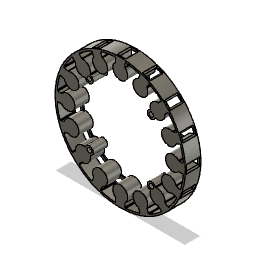
ball_syahei_20221011 v1 (Autodesk Fusion 360 design; units mm, degrees)
Autodesk Fusion 360 part; units mm, degrees
(part 1 of 2)
sketch "スケッチ1" plane through (0, 0, 0) normal (0, 0, 1) x (1, 0, 0)
  line L0 (-2.25, 51.3973) -> (-2.25, 46.9371)
  line L1 (2.25, 51.3973) -> (2.25, 46.9371)
  arc A0 (-2.6591, 46.1303) -> (2.6591, 46.1303) centre (0, 42.5) ccw
  arc A1 (2.25, 46.9371) -> (2.6591, 46.1303) centre (3.25, 46.9371) ccw
  arc A2 (-2.6591, 46.1303) -> (-2.25, 46.9371) centre (-3.25, 46.9371) ccw
  arc A3 (3.3131, 52.3954) -> (2.25, 51.3973) centre (3.25, 51.3973) ccw
  arc A4 (-2.25, 51.3973) -> (-3.3131, 52.3954) centre (-3.25, 51.3973) ccw
  line L2 (3.75, 47.4181) -> (3.75, 50.3208)
  line L3 (-3.75, 50.3208) -> (-3.75, 47.4181)
  arc A5 (-3.9231, 47.0398) -> (3.9231, 47.0398) centre (0, 42.5) ccw
  arc A6 (-3.75, 50.3208) -> (-4.2921, 50.8191) centre (-4.25, 50.3208) ccw
  arc A7 (4.2921, 50.8191) -> (3.75, 50.3208) centre (4.25, 50.3208) ccw
  arc A8 (-3.9231, 47.0398) -> (-3.75, 47.4181) centre (-4.25, 47.4181) ccw
  arc A9 (3.75, 47.4181) -> (3.9231, 47.0398) centre (4.25, 47.4181) ccw
  arc A10 (-15.4823, 48.5932) -> (-15.7924, 47.9255) centre (-15.3305, 48.1168) ccw
  arc A11 (-22.7215, 45.0553) -> (-23.413, 45.3082) centre (-23.1834, 44.864) ccw
  line L4 (-22.7215, 45.0553) -> (-21.6107, 42.3735)
  arc A12 (-21.6258, 41.9578) -> (-21.6107, 42.3735) centre (-22.0726, 42.1822) ccw
  arc A13 (-21.6258, 41.9578) -> (-14.3769, 44.9604) centre (-16.264, 39.2649) ccw
  arc A14 (-14.6816, 45.2437) -> (-14.3769, 44.9604) centre (-14.2196, 45.435) ccw
  line L5 (-14.6816, 45.2437) -> (-15.7924, 47.9255)
  line L6 (-17.5902, 48.346) -> (-15.8833, 44.2252)
  arc A15 (-15.8833, 44.2252) -> (-15.1966, 43.6365) centre (-14.9594, 44.6079) ccw
  arc A16 (-20.11, 41.6013) -> (-15.1966, 43.6365) centre (-16.264, 39.2649) ccw
  arc A17 (-20.11, 41.6013) -> (-20.0408, 42.5032) centre (-20.9646, 42.1205) ccw
  line L7 (-21.7476, 46.6239) -> (-20.0408, 42.5032)
  arc A18 (-21.7476, 46.6239) -> (-23.1117, 47.1391) centre (-22.6715, 46.2412) ccw
  arc A19 (-16.9899, 49.6749) -> (-17.5902, 48.346) centre (-16.6663, 48.7287) ccw
  arc A20 (-32.8996, 38.9695) -> (-32.9306, 38.2339) centre (-32.577, 38.5874) ccw
  arc A21 (-38.2339, 32.9306) -> (-38.9695, 32.8996) centre (-38.5874, 32.577) ccw
  line L8 (-38.2339, 32.9306) -> (-36.1813, 30.878)
  arc A22 (-36.0362, 30.4881) -> (-36.1813, 30.878) centre (-36.5348, 30.5244) ccw
  arc A23 (-30.878, 36.1813) -> (-30.4881, 36.0362) centre (-30.5244, 36.5348) ccw
  line L9 (-30.878, 36.1813) -> (-32.9306, 38.2339)
  line L10 (-34.7524, 37.9344) -> (-31.5985, 34.7805)
  arc A24 (-31.5985, 34.7805) -> (-30.7388, 34.4993) centre (-30.8914, 35.4876) ccw
  arc A25 (-34.4993, 30.7388) -> (-30.7388, 34.4993) centre (-30.052, 30.052) ccw
  arc A26 (-34.4993, 30.7388) -> (-34.7805, 31.5985) centre (-35.4876, 30.8914) ccw
  line L11 (-37.9344, 34.7524) -> (-34.7805, 31.5985)
  arc A27 (-37.9344, 34.7524) -> (-39.3918, 34.7064) centre (-38.6415, 34.0453) ccw
  arc A28 (-34.7064, 39.3918) -> (-34.7524, 37.9344) centre (-34.0453, 38.6415) ccw
  arc A29 (-45.3082, 23.413) -> (-45.0553, 22.7215) centre (-44.864, 23.1834) ccw
  arc A30 (-47.9255, 15.7924) -> (-48.5932, 15.4823) centre (-48.1168, 15.3305) ccw
  line L12 (-47.9255, 15.7924) -> (-45.2437, 14.6816)
  arc A31 (-44.9604, 14.3769) -> (-45.2437, 14.6816) centre (-45.435, 14.2196) ccw
  arc A32 (-44.9604, 14.3769) -> (-41.9578, 21.6258) centre (-39.2649, 16.264) ccw
  arc A33 (-42.3735, 21.6107) -> (-41.9578, 21.6258) centre (-42.1822, 22.0726) ccw
  line L13 (-42.3735, 21.6107) -> (-45.0553, 22.7215)
  line L14 (-46.6239, 21.7476) -> (-42.5032, 20.0408)
  arc A34 (-42.5032, 20.0408) -> (-41.6013, 20.11) centre (-42.1205, 20.9646) ccw
  arc A35 (-43.6365, 15.1966) -> (-41.6013, 20.11) centre (-39.2649, 16.264) ccw
  arc A36 (-43.6365, 15.1966) -> (-44.2252, 15.8833) centre (-44.6079, 14.9594) ccw
  line L15 (-48.346, 17.5902) -> (-44.2252, 15.8833)
  arc A37 (-48.346, 17.5902) -> (-49.6749, 16.9899) centre (-48.7287, 16.6663) ccw
  arc A38 (-47.1391, 23.1117) -> (-46.6239, 21.7476) centre (-46.2412, 22.6715) ccw
  arc A39 (-50.8191, 4.2921) -> (-50.3208, 3.75) centre (-50.3208, 4.25) ccw
  arc A40 (-50.3208, -3.75) -> (-50.8191, -4.2921) centre (-50.3208, -4.25) ccw
  line L16 (-50.3208, -3.75) -> (-47.4181, -3.75)
  arc A41 (-47.0398, -3.9231) -> (-47.4181, -3.75) centre (-47.4181, -4.25) ccw
  arc A42 (-47.0398, -3.9231) -> (-47.0398, 3.9231) centre (-42.5, 0) ccw
  arc A43 (-47.4181, 3.75) -> (-47.0398, 3.9231) centre (-47.4181, 4.25) ccw
  line L17 (-47.4181, 3.75) -> (-50.3208, 3.75)
  line L18 (-51.3973, 2.25) -> (-46.9371, 2.25)
  arc A44 (-46.9371, 2.25) -> (-46.1303, 2.6591) centre (-46.9371, 3.25) ccw
  arc A45 (-46.1303, -2.6591) -> (-46.1303, 2.6591) centre (-42.5, 0) ccw
  arc A46 (-46.1303, -2.6591) -> (-46.9371, -2.25) centre (-46.9371, -3.25) ccw
  line L19 (-51.3973, -2.25) -> (-46.9371, -2.25)
  arc A47 (-51.3973, -2.25) -> (-52.3954, -3.3131) centre (-51.3973, -3.25) ccw
  arc A48 (-52.3954, 3.3131) -> (-51.3973, 2.25) centre (-51.3973, 3.25) ccw
  arc A49 (-48.5932, -15.4823) -> (-47.9255, -15.7924) centre (-48.1168, -15.3305) ccw
  arc A50 (-45.0553, -22.7215) -> (-45.3082, -23.413) centre (-44.864, -23.1834) ccw
  line L20 (-45.0553, -22.7215) -> (-42.3735, -21.6107)
  arc A51 (-41.9578, -21.6258) -> (-42.3735, -21.6107) centre (-42.1822, -22.0726) ccw
  arc A52 (-41.9578, -21.6258) -> (-44.9604, -14.3769) centre (-39.2649, -16.264) ccw
  arc A53 (-45.2437, -14.6816) -> (-44.9604, -14.3769) centre (-45.435, -14.2196) ccw
  line L21 (-45.2437, -14.6816) -> (-47.9255, -15.7924)
  line L22 (-48.346, -17.5902) -> (-44.2252, -15.8833)
  arc A54 (-44.2252, -15.8833) -> (-43.6365, -15.1966) centre (-44.6079, -14.9594) ccw
  arc A55 (-41.6013, -20.11) -> (-43.6365, -15.1966) centre (-39.2649, -16.264) ccw
  arc A56 (-41.6013, -20.11) -> (-42.5032, -20.0408) centre (-42.1205, -20.9646) ccw
  line L23 (-46.6239, -21.7476) -> (-42.5032, -20.0408)
  arc A57 (-46.6239, -21.7476) -> (-47.1391, -23.1117) centre (-46.2412, -22.6715) ccw
  arc A58 (-49.6749, -16.9899) -> (-48.346, -17.5902) centre (-48.7287, -16.6663) ccw
  arc A59 (-38.9695, -32.8996) -> (-38.2339, -32.9306) centre (-38.5874, -32.577) ccw
  arc A60 (-32.9306, -38.2339) -> (-32.8996, -38.9695) centre (-32.577, -38.5874) ccw
  line L24 (-32.9306, -38.2339) -> (-30.878, -36.1813)
  arc A61 (-30.4881, -36.0362) -> (-30.878, -36.1813) centre (-30.5244, -36.5348) ccw
  arc A62 (-36.1813, -30.878) -> (-36.0362, -30.4881) centre (-36.5348, -30.5244) ccw
  line L25 (-36.1813, -30.878) -> (-38.2339, -32.9306)
  line L26 (-37.9344, -34.7524) -> (-34.7805, -31.5985)
  arc A63 (-34.7805, -31.5985) -> (-34.4993, -30.7388) centre (-35.4876, -30.8914) ccw
  arc A64 (-30.7388, -34.4993) -> (-34.4993, -30.7388) centre (-30.052, -30.052) ccw
  arc A65 (-30.7388, -34.4993) -> (-31.5985, -34.7805) centre (-30.8914, -35.4876) ccw
  line L27 (-34.7524, -37.9344) -> (-31.5985, -34.7805)
  arc A66 (-34.7524, -37.9344) -> (-34.7064, -39.3918) centre (-34.0453, -38.6415) ccw
  arc A67 (-39.3918, -34.7064) -> (-37.9344, -34.7524) centre (-38.6415, -34.0453) ccw
  arc A68 (-23.413, -45.3082) -> (-22.7215, -45.0553) centre (-23.1834, -44.864) ccw
  arc A69 (-15.7924, -47.9255) -> (-15.4823, -48.5932) centre (-15.3305, -48.1168) ccw
  line L28 (-15.7924, -47.9255) -> (-14.6816, -45.2437)
  arc A70 (-14.3769, -44.9604) -> (-14.6816, -45.2437) centre (-14.2196, -45.435) ccw
  arc A71 (-14.3769, -44.9604) -> (-21.6258, -41.9578) centre (-16.264, -39.2649) ccw
  arc A72 (-21.6107, -42.3735) -> (-21.6258, -41.9578) centre (-22.0726, -42.1822) ccw
  line L29 (-21.6107, -42.3735) -> (-22.7215, -45.0553)
  line L30 (-21.7476, -46.6239) -> (-20.0408, -42.5032)
  arc A73 (-20.0408, -42.5032) -> (-20.11, -41.6013) centre (-20.9646, -42.1205) ccw
  arc A74 (-15.1966, -43.6365) -> (-20.11, -41.6013) centre (-16.264, -39.2649) ccw
  arc A75 (-15.1966, -43.6365) -> (-15.8833, -44.2252) centre (-14.9594, -44.6079) ccw
  line L31 (-17.5902, -48.346) -> (-15.8833, -44.2252)
  arc A76 (-17.5902, -48.346) -> (-16.9899, -49.6749) centre (-16.6663, -48.7287) ccw
  arc A77 (-23.1117, -47.1391) -> (-21.7476, -46.6239) centre (-22.6715, -46.2412) ccw
  arc A78 (-4.2921, -50.8191) -> (-3.75, -50.3208) centre (-4.25, -50.3208) ccw
  arc A79 (3.75, -50.3208) -> (4.2921, -50.8191) centre (4.25, -50.3208) ccw
  line L32 (3.75, -50.3208) -> (3.75, -47.4181)
  arc A80 (3.9231, -47.0398) -> (3.75, -47.4181) centre (4.25, -47.4181) ccw
  arc A81 (3.9231, -47.0398) -> (-3.9231, -47.0398) centre (0, -42.5) ccw
  arc A82 (-3.75, -47.4181) -> (-3.9231, -47.0398) centre (-4.25, -47.4181) ccw
  line L33 (-3.75, -47.4181) -> (-3.75, -50.3208)
  line L34 (-2.25, -51.3973) -> (-2.25, -46.9371)
  arc A83 (-2.25, -46.9371) -> (-2.6591, -46.1303) centre (-3.25, -46.9371) ccw
  arc A84 (2.6591, -46.1303) -> (-2.6591, -46.1303) centre (0, -42.5) ccw
  arc A85 (2.6591, -46.1303) -> (2.25, -46.9371) centre (3.25, -46.9371) ccw
  line L35 (2.25, -51.3973) -> (2.25, -46.9371)
  arc A86 (2.25, -51.3973) -> (3.3131, -52.3954) centre (3.25, -51.3973) ccw
  arc A87 (-3.3131, -52.3954) -> (-2.25, -51.3973) centre (-3.25, -51.3973) ccw
  arc A88 (15.4823, -48.5932) -> (15.7924, -47.9255) centre (15.3305, -48.1168) ccw
  arc A89 (22.7215, -45.0553) -> (23.413, -45.3082) centre (23.1834, -44.864) ccw
  line L36 (22.7215, -45.0553) -> (21.6107, -42.3735)
  arc A90 (21.6258, -41.9578) -> (21.6107, -42.3735) centre (22.0726, -42.1822) ccw
  arc A91 (21.6258, -41.9578) -> (14.3769, -44.9604) centre (16.264, -39.2649) ccw
  arc A92 (14.6816, -45.2437) -> (14.3769, -44.9604) centre (14.2196, -45.435) ccw
  line L37 (14.6816, -45.2437) -> (15.7924, -47.9255)
  line L38 (17.5902, -48.346) -> (15.8833, -44.2252)
  arc A93 (15.8833, -44.2252) -> (15.1966, -43.6365) centre (14.9594, -44.6079) ccw
  arc A94 (20.11, -41.6013) -> (15.1966, -43.6365) centre (16.264, -39.2649) ccw
  arc A95 (20.11, -41.6013) -> (20.0408, -42.5032) centre (20.9646, -42.1205) ccw
  line L39 (21.7476, -46.6239) -> (20.0408, -42.5032)
  arc A96 (21.7476, -46.6239) -> (23.1117, -47.1391) centre (22.6715, -46.2412) ccw
  arc A97 (16.9899, -49.6749) -> (17.5902, -48.346) centre (16.6663, -48.7287) ccw
  arc A98 (32.8996, -38.9695) -> (32.9306, -38.2339) centre (32.577, -38.5874) ccw
  arc A99 (38.2339, -32.9306) -> (38.9695, -32.8996) centre (38.5874, -32.577) ccw
  line L40 (38.2339, -32.9306) -> (36.1813, -30.878)
  arc A100 (36.0362, -30.4881) -> (36.1813, -30.878) centre (36.5348, -30.5244) ccw
  arc A101 (30.878, -36.1813) -> (30.4881, -36.0362) centre (30.5244, -36.5348) ccw
  line L41 (30.878, -36.1813) -> (32.9306, -38.2339)
  line L42 (34.7524, -37.9344) -> (31.5985, -34.7805)
  arc A102 (31.5985, -34.7805) -> (30.7388, -34.4993) centre (30.8914, -35.4876) ccw
  arc A103 (34.4993, -30.7388) -> (30.7388, -34.4993) centre (30.052, -30.052) ccw
  arc A104 (34.4993, -30.7388) -> (34.7805, -31.5985) centre (35.4876, -30.8914) ccw
  line L43 (37.9344, -34.7524) -> (34.7805, -31.5985)
  arc A105 (37.9344, -34.7524) -> (39.3918, -34.7064) centre (38.6415, -34.0453) ccw
  arc A106 (34.7064, -39.3918) -> (34.7524, -37.9344) centre (34.0453, -38.6415) ccw
  arc A107 (45.3082, -23.413) -> (45.0553, -22.7215) centre (44.864, -23.1834) ccw
  arc A108 (47.9255, -15.7924) -> (48.5932, -15.4823) centre (48.1168, -15.3305) ccw
  line L44 (47.9255, -15.7924) -> (45.2437, -14.6816)
  arc A109 (44.9604, -14.3769) -> (45.2437, -14.6816) centre (45.435, -14.2196) ccw
  arc A110 (44.9604, -14.3769) -> (41.9578, -21.6258) centre (39.2649, -16.264) ccw
  arc A111 (42.3735, -21.6107) -> (41.9578, -21.6258) centre (42.1822, -22.0726) ccw
  line L45 (42.3735, -21.6107) -> (45.0553, -22.7215)
  line L46 (46.6239, -21.7476) -> (42.5032, -20.0408)
  arc A112 (42.5032, -20.0408) -> (41.6013, -20.11) centre (42.1205, -20.9646) ccw
  arc A113 (43.6365, -15.1966) -> (41.6013, -20.11) centre (39.2649, -16.264) ccw
  arc A114 (43.6365, -15.1966) -> (44.2252, -15.8833) centre (44.6079, -14.9594) ccw
  line L47 (48.346, -17.5902) -> (44.2252, -15.8833)
  arc A115 (48.346, -17.5902) -> (49.6749, -16.9899) centre (48.7287, -16.6663) ccw
  arc A116 (47.1391, -23.1117) -> (46.6239, -21.7476) centre (46.2412, -22.6715) ccw
  arc A117 (50.8191, -4.2921) -> (50.3208, -3.75) centre (50.3208, -4.25) ccw
  arc A118 (50.3208, 3.75) -> (50.8191, 4.2921) centre (50.3208, 4.25) ccw
  line L48 (50.3208, 3.75) -> (47.4181, 3.75)
  arc A119 (47.0398, 3.9231) -> (47.4181, 3.75) centre (47.4181, 4.25) ccw
  arc A120 (47.0398, 3.9231) -> (47.0398, -3.9231) centre (42.5, 0) ccw
  arc A121 (47.4181, -3.75) -> (47.0398, -3.9231) centre (47.4181, -4.25) ccw
  line L49 (47.4181, -3.75) -> (50.3208, -3.75)
  line L50 (51.3973, -2.25) -> (46.9371, -2.25)
  arc A122 (46.9371, -2.25) -> (46.1303, -2.6591) centre (46.9371, -3.25) ccw
  arc A123 (46.1303, 2.6591) -> (46.1303, -2.6591) centre (42.5, 0) ccw
  arc A124 (46.1303, 2.6591) -> (46.9371, 2.25) centre (46.9371, 3.25) ccw
  line L51 (51.3973, 2.25) -> (46.9371, 2.25)
  arc A125 (51.3973, 2.25) -> (52.3954, 3.3131) centre (51.3973, 3.25) ccw
  arc A126 (52.3954, -3.3131) -> (51.3973, -2.25) centre (51.3973, -3.25) ccw
  arc A127 (48.5932, 15.4823) -> (47.9255, 15.7924) centre (48.1168, 15.3305) ccw
  arc A128 (45.0553, 22.7215) -> (45.3082, 23.413) centre (44.864, 23.1834) ccw
  line L52 (45.0553, 22.7215) -> (42.3735, 21.6107)
  arc A129 (41.9578, 21.6258) -> (42.3735, 21.6107) centre (42.1822, 22.0726) ccw
  arc A130 (41.9578, 21.6258) -> (44.9604, 14.3769) centre (39.2649, 16.264) ccw
  arc A131 (45.2437, 14.6816) -> (44.9604, 14.3769) centre (45.435, 14.2196) ccw
  line L53 (45.2437, 14.6816) -> (47.9255, 15.7924)
  line L54 (48.346, 17.5902) -> (44.2252, 15.8833)
  arc A132 (44.2252, 15.8833) -> (43.6365, 15.1966) centre (44.6079, 14.9594) ccw
  arc A133 (41.6013, 20.11) -> (43.6365, 15.1966) centre (39.2649, 16.264) ccw
  arc A134 (41.6013, 20.11) -> (42.5032, 20.0408) centre (42.1205, 20.9646) ccw
  line L55 (46.6239, 21.7476) -> (42.5032, 20.0408)
  arc A135 (46.6239, 21.7476) -> (47.1391, 23.1117) centre (46.2412, 22.6715) ccw
  arc A136 (49.6749, 16.9899) -> (48.346, 17.5902) centre (48.7287, 16.6663) ccw
  arc A137 (38.9695, 32.8996) -> (38.2339, 32.9306) centre (38.5874, 32.577) ccw
  arc A138 (32.9306, 38.2339) -> (32.8996, 38.9695) centre (32.577, 38.5874) ccw
  line L56 (32.9306, 38.2339) -> (30.878, 36.1813)
  arc A139 (30.4881, 36.0362) -> (30.878, 36.1813) centre (30.5244, 36.5348) ccw
  arc A140 (36.1813, 30.878) -> (36.0362, 30.4881) centre (36.5348, 30.5244) ccw
  line L57 (36.1813, 30.878) -> (38.2339, 32.9306)
  line L58 (37.9344, 34.7524) -> (34.7805, 31.5985)
  arc A141 (34.7805, 31.5985) -> (34.4993, 30.7388) centre (35.4876, 30.8914) ccw
  arc A142 (30.7388, 34.4993) -> (34.4993, 30.7388) centre (30.052, 30.052) ccw
  arc A143 (30.7388, 34.4993) -> (31.5985, 34.7805) centre (30.8914, 35.4876) ccw
  line L59 (34.7524, 37.9344) -> (31.5985, 34.7805)
  arc A144 (34.7524, 37.9344) -> (34.7064, 39.3918) centre (34.0453, 38.6415) ccw
  arc A145 (39.3918, 34.7064) -> (37.9344, 34.7524) centre (38.6415, 34.0453) ccw
  arc A146 (23.413, 45.3082) -> (22.7215, 45.0553) centre (23.1834, 44.864) ccw
  arc A147 (15.7924, 47.9255) -> (15.4823, 48.5932) centre (15.3305, 48.1168) ccw
  line L60 (15.7924, 47.9255) -> (14.6816, 45.2437)
  arc A148 (14.3769, 44.9604) -> (14.6816, 45.2437) centre (14.2196, 45.435) ccw
  arc A149 (14.3769, 44.9604) -> (21.6258, 41.9578) centre (16.264, 39.2649) ccw
  arc A150 (21.6107, 42.3735) -> (21.6258, 41.9578) centre (22.0726, 42.1822) ccw
  line L61 (21.6107, 42.3735) -> (22.7215, 45.0553)
  line L62 (21.7476, 46.6239) -> (20.0408, 42.5032)
  arc A151 (20.0408, 42.5032) -> (20.11, 41.6013) centre (20.9646, 42.1205) ccw
  arc A152 (15.1966, 43.6365) -> (20.11, 41.6013) centre (16.264, 39.2649) ccw
  arc A153 (15.1966, 43.6365) -> (15.8833, 44.2252) centre (14.9594, 44.6079) ccw
  line L63 (17.5902, 48.346) -> (15.8833, 44.2252)
  arc A154 (17.5902, 48.346) -> (16.9899, 49.6749) centre (16.6663, 48.7287) ccw
  arc A155 (23.1117, 47.1391) -> (21.7476, 46.6239) centre (22.6715, 46.2412) ccw
  arc A156 (-3.3131, 52.3954) -> (-16.9899, 49.6749) centre (0, 0) ccw
  arc A157 (-4.2921, 50.8191) -> (-15.4823, 48.5932) centre (0, 0) ccw
  arc A158 (-23.1117, 47.1391) -> (-34.7064, 39.3918) centre (0, 0) ccw
  arc A159 (-23.413, 45.3082) -> (-32.8996, 38.9695) centre (0, 0) ccw
  arc A160 (-39.3918, 34.7064) -> (-47.1391, 23.1117) centre (0, 0) ccw
  arc A161 (-38.9695, 32.8996) -> (-45.3082, 23.413) centre (0, 0) ccw
  arc A162 (-49.6749, 16.9899) -> (-52.3954, 3.3131) centre (0, 0) ccw
  arc A163 (-48.5932, 15.4823) -> (-50.8191, 4.2921) centre (0, 0) ccw
  arc A164 (-52.3954, -3.3131) -> (-49.6749, -16.9899) centre (0, 0) ccw
  arc A165 (-50.8191, -4.2921) -> (-48.5932, -15.4823) centre (0, 0) ccw
  arc A166 (-47.1391, -23.1117) -> (-39.3918, -34.7064) centre (0, 0) ccw
  arc A167 (-45.3082, -23.413) -> (-38.9695, -32.8996) centre (0, 0) ccw
  arc A168 (-34.7064, -39.3918) -> (-23.1117, -47.1391) centre (0, 0) ccw
  arc A169 (-32.8996, -38.9695) -> (-23.413, -45.3082) centre (0, 0) ccw
  arc A170 (-16.9899, -49.6749) -> (-3.3131, -52.3954) centre (0, 0) ccw
  arc A171 (-15.4823, -48.5932) -> (-4.2921, -50.8191) centre (0, 0) ccw
  arc A172 (3.3131, -52.3954) -> (16.9899, -49.6749) centre (0, 0) ccw
  arc A173 (4.2921, -50.8191) -> (15.4823, -48.5932) centre (0, 0) ccw
  arc A174 (23.1117, -47.1391) -> (34.7064, -39.3918) centre (0, 0) ccw
  arc A175 (23.413, -45.3082) -> (32.8996, -38.9695) centre (0, 0) ccw
  arc A176 (39.3918, -34.7064) -> (47.1391, -23.1117) centre (0, 0) ccw
  arc A177 (38.9695, -32.8996) -> (45.3082, -23.413) centre (0, 0) ccw
  arc A178 (49.6749, -16.9899) -> (52.3954, -3.3131) centre (0, 0) ccw
  arc A179 (48.5932, -15.4823) -> (50.8191, -4.2921) centre (0, 0) ccw
  arc A180 (52.3954, 3.3131) -> (49.6749, 16.9899) centre (0, 0) ccw
  arc A181 (50.8191, 4.2921) -> (48.5932, 15.4823) centre (0, 0) ccw
  arc A182 (47.1391, 23.1117) -> (39.3918, 34.7064) centre (0, 0) ccw
  arc A183 (45.3082, 23.413) -> (38.9695, 32.8996) centre (0, 0) ccw
  arc A184 (34.7064, 39.3918) -> (23.1117, 47.1391) centre (0, 0) ccw
  arc A185 (32.8996, 38.9695) -> (23.413, 45.3082) centre (0, 0) ccw
  arc A186 (16.9899, 49.6749) -> (3.3131, 52.3954) centre (0, 0) ccw
  arc A187 (15.4823, 48.5932) -> (4.2921, 50.8191) centre (0, 0) ccw
  circle A188 centre (-25, 25) radius 1.75
  line L64 (0, 0) -> (-25, 0)
  line L65 (0, 0) -> (0, 25)
  arc A189 (-28.0588, 23.9018) -> (-23.9018, 28.0588) centre (-25, 25) ccw
  arc A190 (-36.0362, 30.4881) -> (-28.6466, 24.219) centre (-30.052, 30.052) ccw
  arc A191 (-24.219, 28.6466) -> (-30.4881, 36.0362) centre (-30.052, 30.052) ccw
  arc A192 (-28.0588, 23.9018) -> (-28.6466, 24.219) centre (-28.5294, 23.7329) ccw
  arc A193 (-24.219, 28.6466) -> (-23.9018, 28.0588) centre (-23.7329, 28.5294) ccw
  arc A194 (-28.6466, -24.219) -> (-28.0588, -23.9018) centre (-28.5294, -23.7329) ccw
  arc A195 (-23.9018, -28.0588) -> (-28.0588, -23.9018) centre (-25, -25) ccw
  arc A196 (-23.9018, -28.0588) -> (-24.219, -28.6466) centre (-23.7329, -28.5294) ccw
  circle A197 centre (-25, -25) radius 1.75
  arc A198 (24.219, -28.6466) -> (23.9018, -28.0588) centre (23.7329, -28.5294) ccw
  arc A199 (28.0588, -23.9018) -> (23.9018, -28.0588) centre (25, -25) ccw
  arc A200 (28.0588, -23.9018) -> (28.6466, -24.219) centre (28.5294, -23.7329) ccw
  circle A201 centre (25, -25) radius 1.75
  arc A202 (28.6466, 24.219) -> (28.0588, 23.9018) centre (28.5294, 23.7329) ccw
  arc A203 (23.9018, 28.0588) -> (28.0588, 23.9018) centre (25, 25) ccw
  arc A204 (23.9018, 28.0588) -> (24.219, 28.6466) centre (23.7329, 28.5294) ccw
  circle A205 centre (25, 25) radius 1.75
  arc A206 (30.4881, 36.0362) -> (24.219, 28.6466) centre (30.052, 30.052) ccw
  arc A207 (28.6466, 24.219) -> (36.0362, 30.4881) centre (30.052, 30.052) ccw
  arc A208 (36.0362, -30.4881) -> (28.6466, -24.219) centre (30.052, -30.052) ccw
  arc A209 (24.219, -28.6466) -> (30.4881, -36.0362) centre (30.052, -30.052) ccw
  arc A210 (-30.4881, -36.0362) -> (-24.219, -28.6466) centre (-30.052, -30.052) ccw
  arc A211 (-28.6466, -24.219) -> (-36.0362, -30.4881) centre (-30.052, -30.052) ccw
  dimension "d1" = 105
  dimension "d4" = 9
  dimension "d6" = 4.5
  dimension "d7" = 1
  dimension "d8" = 1
  dimension "d9" = 1
  dimension "d10" = 1
  dimension "d11" = 12
  dimension "d13" = 1.5
  dimension "d14" = 102
  dimension "d15" = 0.5
  dimension "d16" = 0.5
  dimension "d17" = 0.5
  dimension "d18" = 0.5
  dimension "d22" = 360
  dimension "d23" = 3.5
  dimension "d24" = 25
  dimension "d25" = 25
  dimension "d26" = 6.5
  dimension "d27" = 0.5
  dimension "d28" = 0.5
  dimension "d30" = 360
  constraint coincident A156.centre A157.centre
  constraint vertical L0
  constraint parallel L0 L1
  constraint tangent L1 A1
  constraint tangent A0 A1
  constraint tangent L0 A2
  constraint tangent A0 A2
  constraint tangent L1 A3
  constraint tangent A3 A156
  constraint tangent L0 A4
  constraint tangent A4 A156
  constraint concentric A0 A5
  constraint parallel L2 L3
  constraint parallel L1 L2
  constraint tangent L3 A6
  constraint tangent A6 A157
  constraint tangent L2 A7
  constraint tangent A7 A157
  constraint tangent L3 A8
  constraint tangent A5 A8
  constraint tangent L2 A9
  constraint tangent A5 A9
  constraint vertical L65
  constraint concentric A188 A189
  constraint concentric A190 A191
  constraint tangent A189 A192
  constraint tangent A190 A192
  constraint tangent A189 A193
  constraint tangent A191 A193
  constraint concentric A206 A207
  constraint concentric A208 A209
  constraint concentric A210 A211
  measures "d1" diameter of A156
  measures "d4" diameter of A0
  measures "d6" distance of L0 L1
  measures "d7" radius of A1
  measures "d8" radius of A2
  measures "d9" radius of A3
  measures "d10" radius of A4
  measures "d11" diameter of A5
  measures "d13" distance of L1 L2
  measures "d14" diameter of A157
  measures "d15" radius of A6
  measures "d16" radius of A7
  measures "d17" radius of A8
  measures "d18" radius of A9
  measures "d23" diameter of A188
  measures "d24" distance of A188.centre L65
  measures "d25" distance of A188.centre L64
  measures "d26" diameter of A189
  measures "d27" radius of A192
  measures "d28" radius of A193
extrude "押し出し1" add sketch "スケッチ1" against normal blind 9.5 makes body 1
sketch "スケッチ2" plane through (0, 0, 0) normal (0, 0, 1) x (1, 0, 0)
  arc A0 (32.8996, -38.9695) -> (32.9306, -38.2339) centre (32.577, -38.5874) ccw
  arc A1 (36.0362, -30.4881) -> (36.1813, -30.878) centre (36.5348, -30.5244) ccw
  line L0 (42.3735, -21.6107) -> (45.0553, -22.7215)
  line L1 (0, 0) -> (-25, 0)
  arc A2 (48.5932, -15.4823) -> (50.8191, -4.2921) centre (0, 0) ccw
  arc A3 (-50.8191, -4.2921) -> (-48.5932, -15.4823) centre (0, 0) ccw
  arc A4 (21.6107, 42.3735) -> (21.6258, 41.9578) centre (22.0726, 42.1822) ccw
  arc A5 (23.9018, 28.0588) -> (24.219, 28.6466) centre (23.7329, 28.5294) ccw
  arc A6 (-3.9231, 47.0398) -> (3.9231, 47.0398) centre (0, 42.5) ccw
  arc A7 (4.2921, 50.8191) -> (3.75, 50.3208) centre (4.25, 50.3208) ccw
  line L2 (0, 0) -> (0, 25)
  arc A8 (14.3769, 44.9604) -> (14.6816, 45.2437) centre (14.2196, 45.435) ccw
  line L3 (15.7924, 47.9255) -> (14.6816, 45.2437)
  arc A9 (15.4823, 48.5932) -> (4.2921, 50.8191) centre (0, 0) ccw
  arc A10 (-3.9231, 47.0398) -> (-3.75, 47.4181) centre (-4.25, 47.4181) ccw
  line L4 (-3.75, 50.3208) -> (-3.75, 47.4181)
  arc A11 (14.3769, 44.9604) -> (21.6258, 41.9578) centre (16.264, 39.2649) ccw
  arc A12 (3.75, 47.4181) -> (3.9231, 47.0398) centre (4.25, 47.4181) ccw
  arc A13 (15.7924, 47.9255) -> (15.4823, 48.5932) centre (15.3305, 48.1168) ccw
  arc A14 (23.413, 45.3082) -> (22.7215, 45.0553) centre (23.1834, 44.864) ccw
  line L5 (21.6107, 42.3735) -> (22.7215, 45.0553)
  arc A15 (-3.75, 50.3208) -> (-4.2921, 50.8191) centre (-4.25, 50.3208) ccw
  arc A16 (-32.8996, 38.9695) -> (-32.9306, 38.2339) centre (-32.577, 38.5874) ccw
  arc A17 (-28.0588, 23.9018) -> (-23.9018, 28.0588) centre (-25, 25) ccw
  line L6 (-22.7215, 45.0553) -> (-21.6107, 42.3735)
  arc A18 (-23.413, 45.3082) -> (-32.8996, 38.9695) centre (0, 0) ccw
  arc A19 (-21.6258, 41.9578) -> (-21.6107, 42.3735) centre (-22.0726, 42.1822) ccw
  arc A20 (-21.6258, 41.9578) -> (-14.3769, 44.9604) centre (-16.264, 39.2649) ccw
  arc A21 (-24.219, 28.6466) -> (-30.4881, 36.0362) centre (-30.052, 30.052) ccw
  line L7 (-14.6816, 45.2437) -> (-15.7924, 47.9255)
  arc A22 (-14.6816, 45.2437) -> (-14.3769, 44.9604) centre (-14.2196, 45.435) ccw
  arc A23 (-22.7215, 45.0553) -> (-23.413, 45.3082) centre (-23.1834, 44.864) ccw
  arc A24 (-36.0362, 30.4881) -> (-36.1813, 30.878) centre (-36.5348, 30.5244) ccw
  line L8 (-30.878, 36.1813) -> (-32.9306, 38.2339)
  arc A25 (-38.2339, 32.9306) -> (-38.9695, 32.8996) centre (-38.5874, 32.577) ccw
  circle A26 centre (-25, 25) radius 1.75
  arc A27 (-38.9695, 32.8996) -> (-45.3082, 23.413) centre (0, 0) ccw
  arc A28 (-36.0362, 30.4881) -> (-28.6466, 24.219) centre (-30.052, 30.052) ccw
  arc A29 (-4.2921, 50.8191) -> (-15.4823, 48.5932) centre (0, 0) ccw
  arc A30 (-50.3208, -3.75) -> (-50.8191, -4.2921) centre (-50.3208, -4.25) ccw
  line L9 (-50.3208, -3.75) -> (-47.4181, -3.75)
  arc A31 (-45.3082, 23.413) -> (-45.0553, 22.7215) centre (-44.864, 23.1834) ccw
  line L10 (-47.4181, 3.75) -> (-50.3208, 3.75)
  arc A32 (-50.8191, 4.2921) -> (-50.3208, 3.75) centre (-50.3208, 4.25) ccw
  arc A33 (-47.4181, 3.75) -> (-47.0398, 3.9231) centre (-47.4181, 4.25) ccw
  arc A34 (-44.9604, 14.3769) -> (-41.9578, 21.6258) centre (-39.2649, 16.264) ccw
  arc A35 (-15.4823, 48.5932) -> (-15.7924, 47.9255) centre (-15.3305, 48.1168) ccw
  arc A36 (-47.9255, 15.7924) -> (-48.5932, 15.4823) centre (-48.1168, 15.3305) ccw
  arc A37 (-24.219, 28.6466) -> (-23.9018, 28.0588) centre (-23.7329, 28.5294) ccw
  arc A38 (-30.878, 36.1813) -> (-30.4881, 36.0362) centre (-30.5244, 36.5348) ccw
  line L11 (-38.2339, 32.9306) -> (-36.1813, 30.878)
  arc A39 (-42.3735, 21.6107) -> (-41.9578, 21.6258) centre (-42.1822, 22.0726) ccw
  arc A40 (-47.0398, -3.9231) -> (-47.4181, -3.75) centre (-47.4181, -4.25) ccw
  arc A41 (-4.2921, -50.8191) -> (-3.75, -50.3208) centre (-4.25, -50.3208) ccw
  line L12 (30.878, -36.1813) -> (32.9306, -38.2339)
  line L13 (47.9255, -15.7924) -> (45.2437, -14.6816)
  arc A42 (38.9695, -32.8996) -> (45.3082, -23.413) centre (0, 0) ccw
  arc A43 (45.3082, -23.413) -> (45.0553, -22.7215) centre (44.864, -23.1834) ccw
  arc A44 (28.0588, -23.9018) -> (28.6466, -24.219) centre (28.5294, -23.7329) ccw
  arc A45 (36.0362, -30.4881) -> (28.6466, -24.219) centre (30.052, -30.052) ccw
  arc A46 (44.9604, -14.3769) -> (45.2437, -14.6816) centre (45.435, -14.2196) ccw
  arc A47 (30.878, -36.1813) -> (30.4881, -36.0362) centre (30.5244, -36.5348) ccw
  arc A48 (28.6466, 24.219) -> (28.0588, 23.9018) centre (28.5294, 23.7329) ccw
  arc A49 (38.9695, 32.8996) -> (38.2339, 32.9306) centre (38.5874, 32.577) ccw
  line L14 (45.0553, 22.7215) -> (42.3735, 21.6107)
  line L15 (45.2437, 14.6816) -> (47.9255, 15.7924)
  arc A50 (28.6466, 24.219) -> (36.0362, 30.4881) centre (30.052, 30.052) ccw
  arc A51 (45.2437, 14.6816) -> (44.9604, 14.3769) centre (45.435, 14.2196) ccw
  arc A52 (36.1813, 30.878) -> (36.0362, 30.4881) centre (36.5348, 30.5244) ccw
  arc A53 (48.5932, 15.4823) -> (47.9255, 15.7924) centre (48.1168, 15.3305) ccw
  arc A54 (45.3082, 23.413) -> (38.9695, 32.8996) centre (0, 0) ccw
  arc A55 (32.9306, 38.2339) -> (32.8996, 38.9695) centre (32.577, 38.5874) ccw
  line L16 (32.9306, 38.2339) -> (30.878, 36.1813)
  arc A56 (45.0553, 22.7215) -> (45.3082, 23.413) centre (44.864, 23.1834) ccw
  arc A57 (30.4881, 36.0362) -> (30.878, 36.1813) centre (30.5244, 36.5348) ccw
  line L17 (36.1813, 30.878) -> (38.2339, 32.9306)
  arc A58 (-44.9604, 14.3769) -> (-45.2437, 14.6816) centre (-45.435, 14.2196) ccw
  line L18 (-42.3735, 21.6107) -> (-45.0553, 22.7215)
  arc A59 (-28.0588, 23.9018) -> (-28.6466, 24.219) centre (-28.5294, 23.7329) ccw
  arc A60 (30.4881, 36.0362) -> (24.219, 28.6466) centre (30.052, 30.052) ccw
  arc A61 (-48.5932, 15.4823) -> (-50.8191, 4.2921) centre (0, 0) ccw
  line L19 (-47.9255, 15.7924) -> (-45.2437, 14.6816)
  arc A62 (50.8191, 4.2921) -> (48.5932, 15.4823) centre (0, 0) ccw
  circle A63 centre (25, 25) radius 1.75
  arc A64 (-47.0398, -3.9231) -> (-47.0398, 3.9231) centre (-42.5, 0) ccw
  arc A65 (41.9578, 21.6258) -> (44.9604, 14.3769) centre (39.2649, 16.264) ccw
  arc A66 (41.9578, 21.6258) -> (42.3735, 21.6107) centre (42.1822, 22.0726) ccw
  arc A67 (32.8996, 38.9695) -> (23.413, 45.3082) centre (0, 0) ccw
  arc A68 (23.9018, 28.0588) -> (28.0588, 23.9018) centre (25, 25) ccw
  arc A69 (47.0398, 3.9231) -> (47.4181, 3.75) centre (47.4181, 4.25) ccw
  arc A70 (50.8191, -4.2921) -> (50.3208, -3.75) centre (50.3208, -4.25) ccw
  arc A71 (50.3208, 3.75) -> (50.8191, 4.2921) centre (50.3208, 4.25) ccw
  line L20 (47.4181, -3.75) -> (50.3208, -3.75)
  arc A72 (47.4181, -3.75) -> (47.0398, -3.9231) centre (47.4181, -4.25) ccw
  line L21 (50.3208, 3.75) -> (47.4181, 3.75)
  arc A73 (47.0398, 3.9231) -> (47.0398, -3.9231) centre (42.5, 0) ccw
  line L22 (3.75, 47.4181) -> (3.75, 50.3208)
  arc A74 (28.0588, -23.9018) -> (23.9018, -28.0588) centre (25, -25) ccw
  arc A75 (24.219, -28.6466) -> (30.4881, -36.0362) centre (30.052, -30.052) ccw
  arc A76 (42.3735, -21.6107) -> (41.9578, -21.6258) centre (42.1822, -22.0726) ccw
  arc A77 (47.9255, -15.7924) -> (48.5932, -15.4823) centre (48.1168, -15.3305) ccw
  circle A78 centre (25, -25) radius 1.75
  arc A79 (23.413, -45.3082) -> (32.8996, -38.9695) centre (0, 0) ccw
  arc A80 (-3.75, -47.4181) -> (-3.9231, -47.0398) centre (-4.25, -47.4181) ccw
  arc A81 (24.219, -28.6466) -> (23.9018, -28.0588) centre (23.7329, -28.5294) ccw
  arc A82 (14.6816, -45.2437) -> (14.3769, -44.9604) centre (14.2196, -45.435) ccw
  arc A83 (-28.6466, -24.219) -> (-28.0588, -23.9018) centre (-28.5294, -23.7329) ccw
  arc A84 (3.75, -50.3208) -> (4.2921, -50.8191) centre (4.25, -50.3208) ccw
  arc A85 (4.2921, -50.8191) -> (15.4823, -48.5932) centre (0, 0) ccw
  line L23 (22.7215, -45.0553) -> (21.6107, -42.3735)
  line L24 (-3.75, -47.4181) -> (-3.75, -50.3208)
  arc A86 (22.7215, -45.0553) -> (23.413, -45.3082) centre (23.1834, -44.864) ccw
  arc A87 (21.6258, -41.9578) -> (21.6107, -42.3735) centre (22.0726, -42.1822) ccw
  arc A88 (3.9231, -47.0398) -> (-3.9231, -47.0398) centre (0, -42.5) ccw
  arc A89 (-45.0553, -22.7215) -> (-45.3082, -23.413) centre (-44.864, -23.1834) ccw
  arc A90 (-28.6466, -24.219) -> (-36.0362, -30.4881) centre (-30.052, -30.052) ccw
  arc A91 (-41.9578, -21.6258) -> (-42.3735, -21.6107) centre (-42.1822, -22.0726) ccw
  arc A92 (-32.9306, -38.2339) -> (-32.8996, -38.9695) centre (-32.577, -38.5874) ccw
  line L25 (-32.9306, -38.2339) -> (-30.878, -36.1813)
  line L26 (-45.2437, -14.6816) -> (-47.9255, -15.7924)
  line L27 (-36.1813, -30.878) -> (-38.2339, -32.9306)
  line L28 (-45.0553, -22.7215) -> (-42.3735, -21.6107)
  arc A93 (-48.5932, -15.4823) -> (-47.9255, -15.7924) centre (-48.1168, -15.3305) ccw
  arc A94 (-38.9695, -32.8996) -> (-38.2339, -32.9306) centre (-38.5874, -32.577) ccw
  arc A95 (-32.8996, -38.9695) -> (-23.413, -45.3082) centre (0, 0) ccw
  arc A96 (-15.4823, -48.5932) -> (-4.2921, -50.8191) centre (0, 0) ccw
  arc A97 (-45.2437, -14.6816) -> (-44.9604, -14.3769) centre (-45.435, -14.2196) ccw
  line L29 (-15.7924, -47.9255) -> (-14.6816, -45.2437)
  line L30 (-21.6107, -42.3735) -> (-22.7215, -45.0553)
  circle A98 centre (-25, -25) radius 1.75
  arc A99 (-15.7924, -47.9255) -> (-15.4823, -48.5932) centre (-15.3305, -48.1168) ccw
  arc A100 (-14.3769, -44.9604) -> (-14.6816, -45.2437) centre (-14.2196, -45.435) ccw
  arc A101 (-41.9578, -21.6258) -> (-44.9604, -14.3769) centre (-39.2649, -16.264) ccw
  arc A102 (-30.4881, -36.0362) -> (-24.219, -28.6466) centre (-30.052, -30.052) ccw
  arc A103 (-36.1813, -30.878) -> (-36.0362, -30.4881) centre (-36.5348, -30.5244) ccw
  arc A104 (-23.9018, -28.0588) -> (-24.219, -28.6466) centre (-23.7329, -28.5294) ccw
  arc A105 (-45.3082, -23.413) -> (-38.9695, -32.8996) centre (0, 0) ccw
  arc A106 (-30.4881, -36.0362) -> (-30.878, -36.1813) centre (-30.5244, -36.5348) ccw
  arc A107 (-21.6107, -42.3735) -> (-21.6258, -41.9578) centre (-22.0726, -42.1822) ccw
  arc A108 (-23.9018, -28.0588) -> (-28.0588, -23.9018) centre (-25, -25) ccw
  arc A109 (-14.3769, -44.9604) -> (-21.6258, -41.9578) centre (-16.264, -39.2649) ccw
  arc A110 (-23.413, -45.3082) -> (-22.7215, -45.0553) centre (-23.1834, -44.864) ccw
  line L31 (38.2339, -32.9306) -> (36.1813, -30.878)
  arc A111 (44.9604, -14.3769) -> (41.9578, -21.6258) centre (39.2649, -16.264) ccw
  arc A112 (38.2339, -32.9306) -> (38.9695, -32.8996) centre (38.5874, -32.577) ccw
  arc A113 (15.4823, -48.5932) -> (15.7924, -47.9255) centre (15.3305, -48.1168) ccw
  line L32 (3.75, -50.3208) -> (3.75, -47.4181)
  arc A114 (3.9231, -47.0398) -> (3.75, -47.4181) centre (4.25, -47.4181) ccw
  line L33 (14.6816, -45.2437) -> (15.7924, -47.9255)
  arc A115 (21.6258, -41.9578) -> (14.3769, -44.9604) centre (16.264, -39.2649) ccw
  circle A116 centre (0, 0) radius 52.5
  dimension "d36" = 360
  dimension "d44" = 12
  dimension "d46" = 102
  dimension "d47" = 0.5
  dimension "d48" = 0.5
  dimension "d49" = 0.5
  dimension "d50" = 0.5
  dimension "d51" = 3.5
  dimension "d52" = 25
  dimension "d53" = 25
  dimension "d54" = 6.5
  dimension "d55" = 0.5
  dimension "d56" = 0.5
  dimension "d57" = 105
  constraint parallel L4 L22
  constraint tangent L4 A15
  constraint tangent A15 A29
  constraint tangent A7 L22
  constraint tangent A7 A29
  constraint tangent A10 L4
  constraint tangent A6 A10
  constraint tangent A12 L22
  constraint tangent A6 A12
  constraint vertical L2
  constraint concentric A17 A26
  constraint concentric A21 A28
  constraint tangent A17 A59
  constraint tangent A28 A59
  constraint tangent A17 A37
  constraint tangent A21 A37
  constraint concentric A50 A60
  constraint concentric A45 A75
  constraint concentric A90 A102
  constraint coincident L1.start A2.centre
  measures "d44" diameter of A6
  measures "d46" diameter of A29
  measures "d47" radius of A15
  measures "d48" radius of A7
  measures "d49" radius of A10
  measures "d50" radius of A12
  measures "d51" diameter of A26
  measures "d52" distance of A17.centre L2
  measures "d53" distance of A17.centre L1
  measures "d54" diameter of A17
  measures "d55" radius of A59
  measures "d56" radius of A37
  measures "d57" diameter of A116
extrude "押し出し2" add sketch "スケッチ2" along normal blind 1 separate body makes body 2